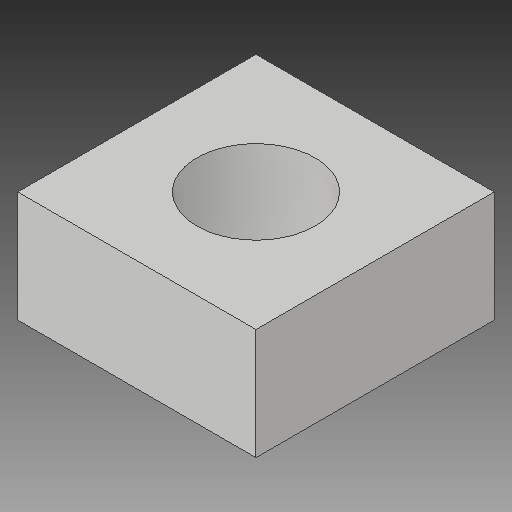
# Autodesk Inventor part: solder_hole
Saved by Autodesk Inventor 2018 (Build 220112000, 112)
## iProperties
Created: 2019-03-04
Part Number: solder_hole
Material: Generic
Document SubType Name: Modeling
Designer: ZEUSLAP
Density: 1 g/cm^3
Appearance: Default
Author: ZEUSLAP
Autodesk Inventor part; units mm, degrees
ref_plane "YZ Plane" through (0, 0, 0) normal (1, 0, 0) x (0, 1, 0)
ref_plane "XZ Plane" through (0, 0, 0) normal (0, 1, 0) x (-1, 0, 0)
ref_plane "XY Plane" through (0, 0, 0) normal (0, 0, 1) x (1, 0, 0)
derived "board.ipt"
sketch "Sketch3" plane through (-0.0909, 21.1322, 23.6321) normal (0, 1, 0) x (1, 0, 0)
  line L0 (0.1364, -2.8636) -> (2.8636, -2.8636)
  line L1 (0.1364, -0.1364) -> (2.8636, -0.1364)
  line L2 (2.8636, -0.1364) -> (2.8636, -2.8636)
  line L3 (2.8636, -2.8636) -> (0.1364, -2.8636)
  line L4 (0.1364, -2.8636) -> (0.1364, -0.1364)
  circle A0 centre (1.5, -1.5) radius 0.6766
  point P0 (0.0909, 23.6321)
  constraints: 10 end point, 1 centre point
extrude "Extrusion1" add sketch "Sketch3" along normal blind 1.27
body "Solid1"
